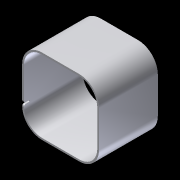
# Autodesk Inventor part: outer
Saved by Autodesk Inventor 2012 (Build 160160000, 160)
## iProperties
Created: 2012-11-10
Part Number: outer
Material: Default
Document SubType Name: Modeling
Designer: SONY
Density: 1 g/cm^3
Author: SONY
Autodesk Inventor part; units mm, degrees
ref_plane "YZ Plane" through (0, 0, 0) normal (1, 0, 0) x (0, 1, 0)
ref_plane "XZ Plane" through (0, 0, 0) normal (0, 1, 0) x (-1, 0, 0)
sketch "Sketch1" plane through (0, 0, 0) normal (0, 0, 1) x (1, 0, 0)
  arc A0 (37.77, -51.7625) -> (57.823, -30.1392) centre (37.77, -31.6525) ccw
  arc A1 (57.88, 4.9774) -> (37.77, 25.0874) centre (37.77, 4.9774) ccw
  arc A2 (-20.11, -31.6525) -> (0, -51.7625) centre (0, -31.6525) ccw
  arc A3 (0, 25.0874) -> (-20.11, 4.9774) centre (0, 4.9774) ccw
  line L0 (37.77, 25.0874) -> (0, 25.0874)
  line L1 (-20.11, -31.6525) -> (-20.11, 4.9774)
  line L2 (57.88, 4.9774) -> (57.88, -31.6525)
  line L3 (38.6468, -51.7625) -> (0, -51.7625)
  line L4 (27.06, -29.8525) -> (27.06, -31.6525) projected
  line L5 (20.48, -29.8525) -> (20.48, -31.8868) projected
  line L6 (5.94, -31.6525) -> (5.94, -29.8525) projected
  line L7 (12.52, -31.6525) -> (12.52, -29.8525) projected
  line L8 (1.8, -23.26) -> (0, -23.26) projected
  line L9 (1.8, -16.68) -> (0, -16.68) projected
  line L10 (0, -8.4695) -> (1.8, -8.4695) projected
  line L11 (0, -2.14) -> (1.8, -2.14) projected
  line L12 (37.77, 23.2874) -> (0, 23.2874) projected
  arc A4 (0, 23.2874) -> (-18.31, 4.9774) centre (0, 4.9774) ccw projected
  line L13 (-18.31, -31.6525) -> (-18.31, 4.9774) projected
  arc A5 (-18.31, -31.6525) -> (0, -49.9625) centre (0, -31.6525) ccw projected
  line L14 (37.77, -49.9625) -> (0, -49.9625) projected
  arc A6 (37.77, -49.9625) -> (56.08, -31.6525) centre (37.77, -31.6525) ccw projected
  line L15 (56.08, 4.9774) -> (56.08, -31.6525) projected
  arc A7 (56.08, 4.9774) -> (37.77, 23.2874) centre (37.77, 4.9774) ccw projected
  line L16 (20.48, -29.8525) -> (12.52, -29.8525) projected
  line L17 (12.52, -31.6525) -> (16.485, -31.6525) projected
  arc A8 (17.985, -33.1525) -> (16.485, -31.6525) centre (16.485, -33.1525) ccw projected
  line L18 (17.985, -36.5025) -> (17.985, -33.1525) projected
  arc A9 (16.485, -38.0025) -> (17.985, -36.5025) centre (16.485, -36.5025) ccw projected
  line L19 (0, -38.0025) -> (16.485, -38.0025) projected
  arc A10 (-1.669, -37.7792) -> (0, -38.0025) centre (0, -31.6525) ccw projected
  arc A11 (-2.3373, -35.2732) -> (-1.669, -37.7792) centre (-1.2747, -36.332) ccw projected
  line L20 (0.942, -31.9822) -> (-2.3373, -35.2732) projected
  arc A12 (2.3363, -31.5782) -> (0.942, -31.9822) centre (2.0045, -33.041) ccw projected
  arc A13 (2.3363, -31.5782) -> (3, -31.6525) centre (3, -28.6525) ccw projected
  line L21 (3, -31.6525) -> (5.94, -31.6525) projected
  line L22 (5.94, -29.8525) -> (4.3, -29.8525) projected
  arc A14 (1.8, -27.3525) -> (4.3, -29.8525) centre (4.3, -27.3525) ccw projected
  line L23 (1.8, -27.3525) -> (1.8, -23.26) projected
  line L24 (0, -28.6525) -> (0, -23.26) projected
  arc A15 (0, -28.6525) -> (0.0741, -29.315) centre (3, -28.6525) ccw projected
  arc A16 (-0.3264, -30.705) -> (0.0741, -29.315) centre (-1.3889, -29.6462) ccw projected
  line L25 (-3.6124, -34.0027) -> (-0.3264, -30.705) projected
  arc A17 (-6.1207, -33.3433) -> (-3.6124, -34.0027) centre (-4.6749, -32.9439) ccw projected
  arc A18 (-6.35, -31.6525) -> (-6.1207, -33.3433) centre (0, -31.6525) ccw projected
  line L26 (-6.35, -15.1) -> (-6.35, -31.6525) projected
  arc A19 (-4.85, -13.6) -> (-6.35, -15.1) centre (-4.85, -15.1) ccw projected
  line L27 (-1.5, -13.6) -> (-4.85, -13.6) projected
  arc A20 (0, -15.1) -> (-1.5, -13.6) centre (-1.5, -15.1) ccw projected
  line L28 (0, -16.68) -> (0, -15.1) projected
  line L29 (1.8, -16.68) -> (1.8, -8.4695) projected
  arc A21 (-1.5, -11.8) -> (0, -10.3) centre (-1.5, -10.3) ccw projected
  line L30 (-4.85, -11.8) -> (-1.5, -11.8) projected
  arc A22 (-6.35, -10.3) -> (-4.85, -11.8) centre (-4.85, -10.3) ccw projected
  line L31 (-6.35, 6.2525) -> (-6.35, -10.3) projected
  arc A23 (-6.1207, 7.9433) -> (-6.35, 6.2525) centre (0, 6.2525) ccw projected
  arc A24 (-3.6124, 8.6027) -> (-6.1207, 7.9433) centre (-4.6749, 7.5439) ccw projected
  line L32 (-0.3264, 5.305) -> (-3.6124, 8.6027) projected
  arc A25 (0.0741, 3.915) -> (-0.3264, 5.305) centre (-1.3889, 4.2462) ccw projected
  arc A26 (0.0741, 3.915) -> (0, 3.2525) centre (3, 3.2525) ccw projected
  line L33 (0, -2.14) -> (0, 3.2525) projected
  line L34 (1.8, -2.14) -> (1.8, 1.9525) projected
  arc A27 (4.3, 4.4525) -> (1.8, 1.9525) centre (4.3, 1.9525) ccw projected
  line L35 (4.3, 4.4525) -> (5.94, 4.4525) projected
  arc A28 (35.97, 1.9525) -> (33.47, 4.4525) centre (33.47, 1.9525) ccw projected
  line L36 (35.97, 1.9525) -> (35.97, -27.3525) projected
  arc A29 (33.47, -29.8525) -> (35.97, -27.3525) centre (33.47, -27.3525) ccw projected
  line L37 (33.47, -29.8525) -> (27.06, -29.8525) projected
  line L38 (27.06, -31.6525) -> (34.77, -31.6525) projected
  arc A30 (34.77, -31.6525) -> (35.4337, -31.5782) centre (34.77, -28.6525) ccw projected
  arc A31 (36.828, -31.9822) -> (35.4337, -31.5782) centre (35.7655, -33.041) ccw projected
  line L39 (40.1073, -35.2732) -> (36.828, -31.9822) projected
  arc A32 (39.439, -37.7792) -> (40.1073, -35.2732) centre (39.0447, -36.332) ccw projected
  arc A33 (37.77, -38.0025) -> (39.439, -37.7792) centre (37.77, -31.6525) ccw projected
  line L40 (21.285, -38.0025) -> (37.77, -38.0025) projected
  arc A34 (19.785, -36.5025) -> (21.285, -38.0025) centre (21.285, -36.5025) ccw projected
  line L41 (19.785, -33.1525) -> (19.785, -36.5025) projected
  arc A35 (20.48, -31.8868) -> (19.785, -33.1525) centre (21.285, -33.1525) ccw projected
  line L42 (37.77, 3.2525) -> (37.77, -10.3) projected
  arc A36 (37.77, 3.2525) -> (37.6959, 3.915) centre (34.77, 3.2525) ccw projected
  arc A37 (38.0964, 5.305) -> (37.6959, 3.915) centre (39.1589, 4.2462) ccw projected
  line L43 (41.3824, 8.6027) -> (38.0964, 5.305) projected
  arc A38 (43.8907, 7.9433) -> (41.3824, 8.6027) centre (42.4449, 7.5439) ccw projected
  arc A39 (44.12, 6.2525) -> (43.8907, 7.9433) centre (37.77, 6.2525) ccw projected
  line L44 (44.12, -10.3) -> (44.12, 6.2525) projected
  arc A40 (42.62, -11.8) -> (44.12, -10.3) centre (42.62, -10.3) ccw projected
  line L45 (39.27, -11.8) -> (42.62, -11.8) projected
  arc A41 (37.77, -10.3) -> (39.27, -11.8) centre (39.27, -10.3) ccw projected
  line L46 (44.12, -31.6525) -> (44.12, -15.1) projected
  arc A42 (43.8907, -33.3433) -> (44.12, -31.6525) centre (37.77, -31.6525) ccw projected
  arc A43 (41.3824, -34.0027) -> (43.8907, -33.3433) centre (42.4449, -32.9439) ccw projected
  line L47 (38.0964, -30.705) -> (41.3824, -34.0027) projected
  arc A44 (37.6959, -29.315) -> (38.0964, -30.705) centre (39.1589, -29.6462) ccw projected
  arc A45 (37.6959, -29.315) -> (37.77, -28.6525) centre (34.77, -28.6525) ccw projected
  line L48 (37.77, -15.1) -> (37.77, -28.6525) projected
  arc A46 (39.27, -13.6) -> (37.77, -15.1) centre (39.27, -15.1) ccw projected
  line L49 (42.62, -13.6) -> (39.27, -13.6) projected
  arc A47 (44.12, -15.1) -> (42.62, -13.6) centre (42.62, -15.1) ccw projected
  arc A48 (35.4337, 6.1782) -> (34.77, 6.2525) centre (34.77, 3.2525) ccw projected
  line L50 (16.485, 6.2525) -> (12.2695, 6.2525) projected
  arc A49 (19.785, 7.7525) -> (20.48, 6.4868) centre (21.285, 7.7525) ccw projected
  line L51 (19.785, 11.1025) -> (19.785, 7.7525) projected
  arc A50 (21.285, 12.6025) -> (19.785, 11.1025) centre (21.285, 11.1025) ccw projected
  line L52 (37.77, 12.6025) -> (21.285, 12.6025) projected
  arc A51 (39.439, 12.3792) -> (37.77, 12.6025) centre (37.77, 6.2525) ccw projected
  arc A52 (40.1073, 9.8732) -> (39.439, 12.3792) centre (39.0447, 10.932) ccw projected
  line L53 (36.828, 6.5822) -> (40.1073, 9.8732) projected
  arc A53 (35.4337, 6.1782) -> (36.828, 6.5822) centre (35.7655, 7.641) ccw projected
  arc A54 (-1.669, 12.3792) -> (-2.3373, 9.8732) centre (-1.2747, 10.932) ccw projected
  arc A55 (0, 12.6025) -> (-1.669, 12.3792) centre (0, 6.2525) ccw projected
  line L54 (16.485, 12.6025) -> (0, 12.6025) projected
  arc A56 (17.985, 11.1025) -> (16.485, 12.6025) centre (16.485, 11.1025) ccw projected
  line L55 (17.985, 7.7525) -> (17.985, 11.1025) projected
  arc A57 (16.485, 6.2525) -> (17.985, 7.7525) centre (16.485, 7.7525) ccw projected
  line L56 (5.94, 6.2525) -> (3, 6.2525) projected
  arc A58 (3, 6.2525) -> (2.3363, 6.1782) centre (3, 3.2525) ccw projected
  arc A59 (0.942, 6.5822) -> (2.3363, 6.1782) centre (2.0045, 7.641) ccw projected
  line L57 (-2.3373, 9.8732) -> (0.942, 6.5822) projected
  line L58 (0, -10.3) -> (0, -8.4695) projected
  line L59 (5.94, 4.4525) -> (5.94, 6.2525) projected
  line L60 (12.2695, 4.4525) -> (12.2695, 6.2525) projected
  line L61 (12.2695, 4.4525) -> (20.48, 4.4525) projected
  line L62 (20.48, 6.4868) -> (20.48, 4.4525) projected
  line L63 (34.77, 6.2525) -> (27.06, 6.2525) projected
  line L64 (27.06, 6.2525) -> (27.06, 4.4525) projected
  line L65 (27.06, 4.4525) -> (33.47, 4.4525) projected
  point P0 (0, 0)
  dimension "d52" = 1.8
  constraints: 9 point on circle, 8 end point, 8 tangent, 4 centre point, 4 coincident, 2 perpendicular, 1 parallel, 1 point on line
  measures "d52" distance between parallel lines of L13 L1
ref_plane "Work Plane1" through (-11.96, -43.6125, -59.69) normal (0, 0, -1) x (0, 1, 0)
extrude "Extrusion1" add sketch "Sketch1" against normal up to surface (59.69 mm away) contours L3 A2 L1 A3 L0 A1 L2 A0
sketch "Sketch4" plane through (37.77, -51.7625, -59.69) normal (0, 0, -1) x (-1, 0, 0)
  line L0 (27.885, 20.11) -> (27.885, 0)
  line L1 (27.885, 0) -> (9.885, 0)
  line L2 (9.885, 0) -> (9.885, 20.11)
  line L3 (37.77, 48.0625) -> (57.88, 48.0625)
  line L4 (57.88, 48.0625) -> (57.88, 30.0625)
  line L5 (57.88, 30.0625) -> (37.77, 30.0625)
  line L6 (27.885, 58.015) -> (27.885, 76.8499)
  line L7 (27.885, 76.8499) -> (9.885, 76.8499)
  line L8 (9.885, 76.8499) -> (9.885, 58.015)
  line L9 (-20.11, 48.0625) -> (0, 48.0625)
  line L10 (0, 30.0625) -> (-20.11, 30.0625)
  line L11 (-20.11, 30.0625) -> (-20.11, 48.0625)
  arc A0 (3, 58.015) -> (0, 55.015) centre (3, 55.015) ccw
  arc A1 (37.77, 55.015) -> (34.77, 58.015) centre (34.77, 55.015) ccw
  arc A2 (34.77, 20.11) -> (37.77, 23.11) centre (34.77, 23.11) ccw
  arc A3 (0, 23.11) -> (3, 20.11) centre (3, 23.11) ccw
  line L12 (0, 76.8499) -> (37.77, 76.8499) projected
  line L13 (3, 20.11) -> (9.885, 20.11)
  line L14 (0, 23.11) -> (0, 30.0625)
  line L15 (27.885, 20.11) -> (34.77, 20.11)
  line L16 (37.77, 23.11) -> (37.77, 30.0625)
  line L17 (37.77, 48.0625) -> (37.77, 55.015)
  line L18 (34.77, 58.015) -> (27.885, 58.015)
  line L19 (9.885, 58.015) -> (3, 58.015)
  line L20 (4.3, 21.91) -> (33.47, 21.91)
  arc A4 (33.47, 21.91) -> (35.97, 24.41) centre (33.47, 24.41) ccw
  line L21 (35.97, 24.41) -> (35.97, 34.0931)
  line L22 (35.97, 34.0931) -> (35.97, 53.715)
  arc A5 (35.97, 53.715) -> (33.47, 56.215) centre (33.47, 53.715) ccw
  line L23 (33.47, 56.215) -> (4.3, 56.215)
  arc A6 (4.3, 56.215) -> (1.8, 53.715) centre (4.3, 53.715) ccw
  line L24 (1.8, 53.715) -> (1.8, 41.6025)
  line L25 (1.8, 41.6025) -> (1.8, 24.41)
  arc A7 (1.8, 24.41) -> (4.3, 21.91) centre (4.3, 24.41) ccw
  line L26 (0, 55.015) -> (0, 48.0625)
  line L27 (-20.11, 20.11) -> (-20.11, 56.7399) projected
  line L28 (37.77, 0) -> (0, 0) projected
  line L29 (57.88, 56.7399) -> (57.88, 20.11) projected
  arc A8 (0.942, 58.3447) -> (2.3363, 57.9407) centre (2.0045, 59.4035) ccw projected
  line L30 (-2.3373, 61.6357) -> (0.942, 58.3447) projected
  arc A9 (-1.669, 64.1417) -> (-2.3373, 61.6357) centre (-1.2747, 62.6945) ccw projected
  arc A10 (0, 64.365) -> (-1.669, 64.1417) centre (0, 58.015) ccw projected
  line L31 (16.485, 64.365) -> (0, 64.365) projected
  arc A11 (17.985, 62.865) -> (16.485, 64.365) centre (16.485, 62.865) ccw projected
  line L32 (17.985, 59.515) -> (17.985, 62.865) projected
  arc A12 (16.485, 58.015) -> (17.985, 59.515) centre (16.485, 59.515) ccw projected
  line L33 (3, 58.015) -> (16.485, 58.015) projected
  arc A13 (3, 58.015) -> (2.3363, 57.9407) centre (3, 55.015) ccw projected
  arc A14 (35.97, 53.715) -> (33.47, 56.215) centre (33.47, 53.715) ccw projected
  line L34 (35.97, 24.41) -> (35.97, 53.715) projected
  arc A15 (33.47, 21.91) -> (35.97, 24.41) centre (33.47, 24.41) ccw projected
  line L35 (4.3, 21.91) -> (33.47, 21.91) projected
  arc A16 (1.8, 24.41) -> (4.3, 21.91) centre (4.3, 24.41) ccw projected
  line L36 (1.8, 53.715) -> (1.8, 24.41) projected
  arc A17 (4.3, 56.215) -> (1.8, 53.715) centre (4.3, 53.715) ccw projected
  line L37 (33.47, 56.215) -> (4.3, 56.215) projected
  arc A18 (-1.5, 39.9625) -> (0, 41.4625) centre (-1.5, 41.4625) ccw projected
  line L38 (-4.85, 39.9625) -> (-1.5, 39.9625) projected
  arc A19 (-6.35, 41.4625) -> (-4.85, 39.9625) centre (-4.85, 41.4625) ccw projected
  line L39 (-6.35, 58.015) -> (-6.35, 41.4625) projected
  arc A20 (-6.1207, 59.7058) -> (-6.35, 58.015) centre (0, 58.015) ccw projected
  arc A21 (-3.6124, 60.3652) -> (-6.1207, 59.7058) centre (-4.6749, 59.3064) ccw projected
  line L40 (-0.3264, 57.0675) -> (-3.6124, 60.3652) projected
  arc A22 (0.0741, 55.6775) -> (-0.3264, 57.0675) centre (-1.3889, 56.0087) ccw projected
  arc A23 (0.0741, 55.6775) -> (0, 55.015) centre (3, 55.015) ccw projected
  line L41 (0, 41.4625) -> (0, 55.015) projected
  arc A24 (39.27, 38.1625) -> (37.77, 36.6625) centre (39.27, 36.6625) ccw projected
  line L42 (42.62, 38.1625) -> (39.27, 38.1625) projected
  arc A25 (44.12, 36.6625) -> (42.62, 38.1625) centre (42.62, 36.6625) ccw projected
  line L43 (44.12, 20.11) -> (44.12, 36.6625) projected
  arc A26 (43.8907, 18.4192) -> (44.12, 20.11) centre (37.77, 20.11) ccw projected
  arc A27 (41.3824, 17.7598) -> (43.8907, 18.4192) centre (42.4449, 18.8186) ccw projected
  line L44 (38.0964, 21.0575) -> (41.3824, 17.7598) projected
  arc A28 (37.6959, 22.4475) -> (38.0964, 21.0575) centre (39.1589, 22.1163) ccw projected
  arc A29 (37.6959, 22.4475) -> (37.77, 23.11) centre (34.77, 23.11) ccw projected
  line L45 (37.77, 36.6625) -> (37.77, 23.11) projected
  arc A30 (0, 36.6625) -> (-1.5, 38.1625) centre (-1.5, 36.6625) ccw projected
  line L46 (0, 23.11) -> (0, 36.6625) projected
  arc A31 (0, 23.11) -> (0.0741, 22.4475) centre (3, 23.11) ccw projected
  arc A32 (-0.3264, 21.0575) -> (0.0741, 22.4475) centre (-1.3889, 22.1163) ccw projected
  line L47 (-3.6124, 17.7598) -> (-0.3264, 21.0575) projected
  arc A33 (-6.1207, 18.4192) -> (-3.6124, 17.7598) centre (-4.6749, 18.8186) ccw projected
  arc A34 (-6.35, 20.11) -> (-6.1207, 18.4192) centre (0, 20.11) ccw projected
  line L48 (-6.35, 36.6625) -> (-6.35, 20.11) projected
  arc A35 (-4.85, 38.1625) -> (-6.35, 36.6625) centre (-4.85, 36.6625) ccw projected
  line L49 (-1.5, 38.1625) -> (-4.85, 38.1625) projected
  arc A36 (38.0964, 57.0675) -> (37.6959, 55.6775) centre (39.1589, 56.0087) ccw projected
  line L50 (41.3824, 60.3652) -> (38.0964, 57.0675) projected
  arc A37 (43.8907, 59.7058) -> (41.3824, 60.3652) centre (42.4449, 59.3064) ccw projected
  arc A38 (44.12, 58.015) -> (43.8907, 59.7058) centre (37.77, 58.015) ccw projected
  line L51 (44.12, 41.4625) -> (44.12, 58.015) projected
  arc A39 (42.62, 39.9625) -> (44.12, 41.4625) centre (42.62, 41.4625) ccw projected
  line L52 (39.27, 39.9625) -> (42.62, 39.9625) projected
  arc A40 (37.77, 41.4625) -> (39.27, 39.9625) centre (39.27, 41.4625) ccw projected
  line L53 (37.77, 55.015) -> (37.77, 41.4625) projected
  arc A41 (37.77, 55.015) -> (37.6959, 55.6775) centre (34.77, 55.015) ccw projected
  arc A42 (35.4337, 57.9407) -> (36.828, 58.3447) centre (35.7655, 59.4035) ccw projected
  arc A43 (35.4337, 57.9407) -> (34.77, 58.015) centre (34.77, 55.015) ccw projected
  line L54 (21.285, 58.015) -> (34.77, 58.015) projected
  arc A44 (19.785, 59.515) -> (21.285, 58.015) centre (21.285, 59.515) ccw projected
  line L55 (19.785, 62.865) -> (19.785, 59.515) projected
  arc A45 (21.285, 64.365) -> (19.785, 62.865) centre (21.285, 62.865) ccw projected
  line L56 (37.77, 64.365) -> (21.285, 64.365) projected
  arc A46 (39.439, 64.1417) -> (37.77, 64.365) centre (37.77, 58.015) ccw projected
  arc A47 (40.1073, 61.6357) -> (39.439, 64.1417) centre (39.0447, 62.6945) ccw projected
  line L57 (36.828, 58.3447) -> (40.1073, 61.6357) projected
  arc A48 (17.985, 18.61) -> (16.485, 20.11) centre (16.485, 18.61) ccw projected
  line L58 (17.985, 15.26) -> (17.985, 18.61) projected
  arc A49 (16.485, 13.76) -> (17.985, 15.26) centre (16.485, 15.26) ccw projected
  line L59 (0, 13.76) -> (16.485, 13.76) projected
  arc A50 (-1.669, 13.9833) -> (0, 13.76) centre (0, 20.11) ccw projected
  arc A51 (-2.3373, 16.4893) -> (-1.669, 13.9833) centre (-1.2747, 15.4305) ccw projected
  line L60 (0.942, 19.7803) -> (-2.3373, 16.4893) projected
  arc A52 (2.3363, 20.1843) -> (0.942, 19.7803) centre (2.0045, 18.7215) ccw projected
  arc A53 (2.3363, 20.1843) -> (3, 20.11) centre (3, 23.11) ccw projected
  line L61 (16.485, 20.11) -> (3, 20.11) projected
  arc A54 (36.828, 19.7803) -> (35.4337, 20.1843) centre (35.7655, 18.7215) ccw projected
  line L62 (40.1073, 16.4893) -> (36.828, 19.7803) projected
  arc A55 (39.439, 13.9833) -> (40.1073, 16.4893) centre (39.0447, 15.4305) ccw projected
  arc A56 (37.77, 13.76) -> (39.439, 13.9833) centre (37.77, 20.11) ccw projected
  line L63 (21.285, 13.76) -> (37.77, 13.76) projected
  arc A57 (19.785, 15.26) -> (21.285, 13.76) centre (21.285, 15.26) ccw projected
  line L64 (19.785, 18.61) -> (19.785, 15.26) projected
  arc A58 (21.285, 20.11) -> (19.785, 18.61) centre (21.285, 18.61) ccw projected
  line L65 (34.77, 20.11) -> (21.285, 20.11) projected
  arc A59 (34.77, 20.11) -> (35.4337, 20.1843) centre (34.77, 23.11) ccw projected
  arc A60 (0, 66.165) -> (-8.15, 58.015) centre (0, 58.015) ccw projected
  line L66 (-8.15, 20.11) -> (-8.15, 58.015) projected
  arc A61 (-8.15, 20.11) -> (0, 11.96) centre (0, 20.11) ccw projected
  line L67 (37.77, 11.96) -> (0, 11.96) projected
  arc A62 (37.77, 11.96) -> (45.92, 20.11) centre (37.77, 20.11) ccw projected
  line L68 (45.92, 58.015) -> (45.92, 20.11) projected
  arc A63 (45.92, 58.015) -> (37.77, 66.165) centre (37.77, 58.015) ccw projected
  line L69 (0, 66.165) -> (37.77, 66.165) projected
  point P0 (37.77, 51.7625)
  dimension "d58" = 18
  dimension "d59" = 8.1
  dimension "d60" = 18
  dimension "d61" = 8.1
  constraints: 52 end point, 24 collinear, 16 point on circle, 14 tangent, 8 centre point, 8 coincident, 5 parallel, 4 perpendicular, 2 horizontal
  measures "d58" distance of L10.end L9.start
  measures "d59" distance between parallel lines of L38 L9
  measures "d60" distance of L0.end L1.end
  measures "d61" distance between parallel lines of L58 L2
extrude "Extrusion4" add sketch "Sketch4" against normal blind 1.8 contours L65 A58 L64 A57 L63 L0 L67 L2 L59 A49 L58 A48 L61 L13 A3 L14 L46 A30 L49 A35 L48 L10 L66 L9 L39 A19 L38 A18 L41 L26 A0 L19 L33 A12 L32 A11 L31 L8 L69 L6 L56 A45 L55 A44 L54 L18 A1 L17 L53 A40 L52 A39 L51 L3 L68 L5 L43 A25 L42 A24 L45 L16 A2 L15 | L0 L63 A57 L64 A58 L65 | L0 L1 L2 L67 | L2 L61 A48 L58 A49 L59 | L68 L3 L4 L5 | L45 A24 L42 A25 L43 L5 | L10 L11 L9 L66 | L51 A39 L52 A40 L53 L3 | L48 A35 L49 A30 L46 L10 | L9 L41 A18 L38 A19 L39 | L69 L8 L7 L6 | L6 L54 A44 L55 A45 L56 | L31 A11 L32 A12 L33 L8
fillet "Fillet2" radius 3.175 8 edges at (37.77, -21.7, -58.79) (27.885, -31.6525, -58.79) (9.885, -31.6525, -58.79) (0, -21.7, -58.79) (0, -3.7, -58.79) (9.885, 6.2525, -58.79) (37.77, -3.7, -58.79) (27.885, 6.2525, -58.79)
sketch "Sketch5" plane through (37.77, -51.7625, -57.89) normal (0, 0, 1) x (1, 0, 0)
  line L0 (-56.08, 48.0625) -> (-40.945, 48.0625) projected
  line L1 (-40.945, 30.0625) -> (-56.08, 30.0625) projected
  line L2 (-43.82, 34.0625) -> (-38.07, 34.0625)
  line L3 (-38.07, 34.0625) -> (-38.07, 30.0625)
  line L4 (-38.07, 30.0625) -> (-43.82, 30.0625)
  line L5 (-43.82, 30.0625) -> (-43.82, 34.0625)
  line L6 (-43.82, 48.0625) -> (-38.07, 48.0625)
  line L7 (-38.07, 48.0625) -> (-38.07, 44.0625)
  line L8 (-38.07, 44.0625) -> (-43.82, 44.0625)
  line L9 (-43.82, 44.0625) -> (-43.82, 48.0625)
  line L10 (-13.885, 14.1275) -> (-13.885, 19.8775)
  line L11 (-13.885, 19.8775) -> (-9.885, 19.8775)
  line L12 (-9.885, 19.8775) -> (-9.885, 14.1275)
  line L13 (-9.885, 14.1275) -> (-13.885, 14.1275)
  line L14 (-27.885, 14.1275) -> (-27.885, 19.8775)
  line L15 (-27.885, 19.8775) -> (-23.885, 19.8775)
  line L16 (-23.885, 19.8775) -> (-23.885, 14.1275)
  line L17 (-23.885, 14.1275) -> (-27.885, 14.1275)
  line L18 (6.05, 44.0625) -> (0.3, 44.0625)
  line L19 (0.3, 44.0625) -> (0.3, 48.0625)
  line L20 (0.3, 48.0625) -> (6.05, 48.0625)
  line L21 (6.05, 48.0625) -> (6.05, 44.0625)
  line L22 (6.05, 30.0625) -> (0.3, 30.0625)
  line L23 (0.3, 30.0625) -> (0.3, 34.0625)
  line L24 (0.3, 34.0625) -> (6.05, 34.0625)
  line L25 (6.05, 34.0625) -> (6.05, 30.0625)
  line L26 (-23.885, 63.9975) -> (-23.885, 58.2475)
  line L27 (-23.885, 58.2475) -> (-27.885, 58.2475)
  line L28 (-27.885, 58.2475) -> (-27.885, 63.9975)
  line L29 (-27.885, 63.9975) -> (-23.885, 63.9975)
  line L30 (-9.885, 63.9975) -> (-9.885, 58.2475)
  line L31 (-9.885, 58.2475) -> (-13.885, 58.2475)
  line L32 (-13.885, 58.2475) -> (-13.885, 63.9975)
  line L33 (-13.885, 63.9975) -> (-9.885, 63.9975)
  line L34 (3.175, 48.0625) -> (18.31, 48.0625) projected
  line L35 (-17.29, 23.18) -> (-17.29, 21.1457) projected
  line L36 (-17.29, 23.18) -> (-25.25, 23.18) projected
  line L37 (-25.25, 21.38) -> (-25.25, 23.18) projected
  line L38 (-25.25, 21.38) -> (-21.285, 21.38) projected
  arc A0 (-19.785, 19.88) -> (-21.285, 21.38) centre (-21.285, 19.88) ccw projected
  line L39 (-19.785, 16.53) -> (-19.785, 19.88) projected
  arc A1 (-21.285, 15.03) -> (-19.785, 16.53) centre (-21.285, 16.53) ccw projected
  line L40 (-37.77, 15.03) -> (-21.285, 15.03) projected
  arc A2 (-39.439, 15.2533) -> (-37.77, 15.03) centre (-37.77, 21.38) ccw projected
  arc A3 (-40.1073, 17.7593) -> (-39.439, 15.2533) centre (-39.0447, 16.7005) ccw projected
  line L41 (-36.828, 21.0503) -> (-40.1073, 17.7593) projected
  arc A4 (-35.4337, 21.4543) -> (-36.828, 21.0503) centre (-35.7655, 19.9915) ccw projected
  arc A5 (-35.4337, 21.4543) -> (-34.77, 20.11) centre (-34.77, 24.38) ccw projected
  line L42 (-34.77, 21.38) -> (-31.83, 21.38) projected
  line L43 (-31.83, 21.38) -> (-31.83, 23.18) projected
  line L44 (-31.83, 23.18) -> (-33.47, 23.18) projected
  arc A6 (-35.97, 24.41) -> (-33.47, 21.91) centre (-33.47, 25.68) ccw projected
  line L45 (-35.97, 24.41) -> (-35.97, 29.7725) projected
  line L46 (-35.97, 29.7725) -> (-37.77, 29.7725) projected
  line L47 (-37.77, 23.11) -> (-37.77, 29.7725) projected
  arc A7 (-37.77, 23.11) -> (-37.6959, 23.7175) centre (-34.77, 24.38) ccw projected
  arc A8 (-38.0964, 22.3275) -> (-37.6959, 23.7175) centre (-39.1589, 23.3863) ccw projected
  line L48 (-41.3824, 19.0298) -> (-38.0964, 22.3275) projected
  arc A9 (-43.8907, 19.6892) -> (-41.3824, 19.0298) centre (-42.4449, 20.0886) ccw projected
  arc A10 (-44.12, 21.38) -> (-43.8907, 19.6892) centre (-37.77, 21.38) ccw projected
  line L49 (-44.12, 37.9325) -> (-44.12, 21.38) projected
  arc A11 (-42.62, 39.4325) -> (-44.12, 37.9325) centre (-42.62, 37.9325) ccw projected
  line L50 (-39.27, 39.4325) -> (-42.62, 39.4325) projected
  arc A12 (-37.77, 37.9325) -> (-39.27, 39.4325) centre (-39.27, 37.9325) ccw projected
  line L51 (-37.77, 36.3525) -> (-37.77, 37.9325) projected
  line L52 (-35.97, 36.3525) -> (-37.77, 36.3525) projected
  line L53 (-35.97, 36.3525) -> (-35.97, 44.563) projected
  line L54 (-37.77, 44.563) -> (-35.97, 44.563) projected
  line L55 (-37.77, 42.7325) -> (-37.77, 44.563) projected
  arc A13 (-39.27, 41.2325) -> (-37.77, 42.7325) centre (-39.27, 42.7325) ccw projected
  line L56 (-42.62, 41.2325) -> (-39.27, 41.2325) projected
  arc A14 (-44.12, 42.7325) -> (-42.62, 41.2325) centre (-42.62, 42.7325) ccw projected
  line L57 (-44.12, 59.285) -> (-44.12, 42.7325) projected
  arc A15 (-43.8907, 60.9758) -> (-44.12, 59.285) centre (-37.77, 59.285) ccw projected
  arc A16 (-41.3824, 61.6352) -> (-43.8907, 60.9758) centre (-42.4449, 60.5764) ccw projected
  line L58 (-38.0964, 58.3375) -> (-41.3824, 61.6352) projected
  arc A17 (-37.6959, 56.9475) -> (-38.0964, 58.3375) centre (-39.1589, 57.2787) ccw projected
  arc A18 (-37.6959, 56.9475) -> (-37.77, 55.015) centre (-34.77, 56.285) ccw projected
  line L59 (-37.77, 50.8925) -> (-37.77, 55.015) projected
  line L60 (-37.77, 50.8925) -> (-35.97, 50.8925) projected
  line L61 (-35.97, 50.8925) -> (-35.97, 53.715) projected
  arc A19 (-33.47, 56.215) -> (-35.97, 53.715) centre (-33.47, 54.985) ccw projected
  line L62 (-33.47, 57.485) -> (-31.83, 57.485) projected
  line L63 (-31.83, 57.485) -> (-31.83, 59.285) projected
  line L64 (-31.83, 59.285) -> (-34.77, 59.285) projected
  arc A20 (-34.77, 58.015) -> (-35.4337, 59.2107) centre (-34.77, 56.285) ccw projected
  arc A21 (-36.828, 59.6147) -> (-35.4337, 59.2107) centre (-35.7655, 60.6735) ccw projected
  line L65 (-40.1073, 62.9057) -> (-36.828, 59.6147) projected
  arc A22 (-39.439, 65.4117) -> (-40.1073, 62.9057) centre (-39.0447, 63.9645) ccw projected
  arc A23 (-37.77, 65.635) -> (-39.439, 65.4117) centre (-37.77, 59.285) ccw projected
  line L66 (-21.285, 65.635) -> (-37.77, 65.635) projected
  arc A24 (-19.785, 64.135) -> (-21.285, 65.635) centre (-21.285, 64.135) ccw projected
  line L67 (-19.785, 60.785) -> (-19.785, 64.135) projected
  arc A25 (-21.285, 59.285) -> (-19.785, 60.785) centre (-21.285, 60.785) ccw projected
  line L68 (-21.285, 59.285) -> (-25.5005, 59.285) projected
  line L69 (-25.5005, 57.485) -> (-25.5005, 59.285) projected
  line L70 (-25.5005, 57.485) -> (-17.29, 57.485) projected
  line L71 (-17.29, 59.5193) -> (-17.29, 57.485) projected
  arc A26 (-17.985, 60.785) -> (-17.29, 59.5193) centre (-16.485, 60.785) ccw projected
  line L72 (-17.985, 64.135) -> (-17.985, 60.785) projected
  arc A27 (-16.485, 65.635) -> (-17.985, 64.135) centre (-16.485, 64.135) ccw projected
  line L73 (0, 65.635) -> (-16.485, 65.635) projected
  arc A28 (1.669, 65.4117) -> (0, 65.635) centre (0, 59.285) ccw projected
  arc A29 (2.3373, 62.9057) -> (1.669, 65.4117) centre (1.2747, 63.9645) ccw projected
  line L74 (-0.942, 59.6147) -> (2.3373, 62.9057) projected
  arc A30 (-2.3363, 59.2107) -> (-0.942, 59.6147) centre (-2.0045, 60.6735) ccw projected
  arc A31 (-2.3363, 59.2107) -> (-3, 58.015) centre (-3, 56.285) ccw projected
  line L75 (-3, 59.285) -> (-10.71, 59.285) projected
  line L76 (-10.71, 59.285) -> (-10.71, 57.485) projected
  line L77 (-10.71, 57.485) -> (-4.3, 57.485) projected
  arc A32 (-1.8, 53.715) -> (-4.3, 56.215) centre (-4.3, 54.985) ccw projected
  line L78 (-1.8, 53.715) -> (-1.8, 24.41) projected
  arc A33 (-4.3, 21.91) -> (-1.8, 24.41) centre (-4.3, 25.68) ccw projected
  line L79 (-4.3, 23.18) -> (-10.71, 23.18) projected
  line L80 (-10.71, 23.18) -> (-10.71, 21.38) projected
  line L81 (-10.71, 21.38) -> (-3, 21.38) projected
  arc A34 (-3, 20.11) -> (-2.3363, 21.4543) centre (-3, 24.38) ccw projected
  arc A35 (-0.942, 21.0503) -> (-2.3363, 21.4543) centre (-2.0045, 19.9915) ccw projected
  line L82 (2.3373, 17.7593) -> (-0.942, 21.0503) projected
  arc A36 (1.669, 15.2533) -> (2.3373, 17.7593) centre (1.2747, 16.7005) ccw projected
  arc A37 (0, 15.03) -> (1.669, 15.2533) centre (0, 21.38) ccw projected
  line L83 (-16.485, 15.03) -> (0, 15.03) projected
  arc A38 (-17.985, 16.53) -> (-16.485, 15.03) centre (-16.485, 16.53) ccw projected
  line L84 (-17.985, 19.88) -> (-17.985, 16.53) projected
  arc A39 (-17.29, 21.1457) -> (-17.985, 19.88) centre (-16.485, 19.88) ccw projected
  line L85 (6.35, 21.38) -> (6.35, 37.9325) projected
  arc A40 (6.1207, 19.6892) -> (6.35, 21.38) centre (0, 21.38) ccw projected
  arc A41 (3.6124, 19.0298) -> (6.1207, 19.6892) centre (4.6749, 20.0886) ccw projected
  line L86 (0.3264, 22.3275) -> (3.6124, 19.0298) projected
  arc A42 (-0.0741, 23.7175) -> (0.3264, 22.3275) centre (1.3889, 23.3863) ccw projected
  arc A43 (-0.0741, 23.7175) -> (0, 23.11) centre (-3, 24.38) ccw projected
  line L87 (0, 37.9325) -> (0, 23.11) projected
  arc A44 (1.5, 39.4325) -> (0, 37.9325) centre (1.5, 37.9325) ccw projected
  line L88 (4.85, 39.4325) -> (1.5, 39.4325) projected
  arc A45 (6.35, 37.9325) -> (4.85, 39.4325) centre (4.85, 37.9325) ccw projected
  line L89 (0, 55.015) -> (0, 42.7325) projected
  arc A46 (0, 55.015) -> (-0.0741, 56.9475) centre (-3, 56.285) ccw projected
  arc A47 (0.3264, 58.3375) -> (-0.0741, 56.9475) centre (1.3889, 57.2787) ccw projected
  line L90 (3.6124, 61.6352) -> (0.3264, 58.3375) projected
  arc A48 (6.1207, 60.9758) -> (3.6124, 61.6352) centre (4.6749, 60.5764) ccw projected
  arc A49 (6.35, 59.285) -> (6.1207, 60.9758) centre (0, 59.285) ccw projected
  line L91 (6.35, 42.7325) -> (6.35, 59.285) projected
  arc A50 (4.85, 41.2325) -> (6.35, 42.7325) centre (4.85, 42.7325) ccw projected
  line L92 (1.5, 41.2325) -> (4.85, 41.2325) projected
  arc A51 (0, 42.7325) -> (1.5, 41.2325) centre (1.5, 42.7325) ccw projected
  line L93 (0, 77.5899) -> (-37.77, 77.5899) projected
  arc A52 (-37.77, 77.5899) -> (-57.35, 58.0099) centre (-37.77, 58.0099) ccw projected
  line L94 (-57.35, 58.0099) -> (-57.35, 21.38) projected
  arc A53 (-57.35, 21.38) -> (-37.77, 1.8) centre (-37.77, 21.38) ccw projected
  line L95 (-37.77, 1.8) -> (0, 1.8) projected
  arc A54 (0, 1.8) -> (19.58, 21.38) centre (0, 21.38) ccw projected
  line L96 (19.58, 21.38) -> (19.58, 58.0099) projected
  arc A55 (19.58, 58.0099) -> (0, 77.5899) centre (0, 58.0099) ccw projected
  point P0 (-55.445, 32.7025)
  point P1 (-37.77, 51.7625)
  point P2 (-18.885, 39.0625)
  point P3 (-21.285, 22.42)
  point P4 (-3, 26.92)
  point P5 (17.675, 50.5025)
  point P6 (-37.77, 50.5025)
  point P7 (-37.77, 32.7025)
  point P8 (-56.08, 30.0625)
  point P9 (18.31, 48.0625)
  point P10 (-40.945, 48.0625)
  dimension "d40" = 360
  dimension "d53" = 4
  dimension "d54" = 4
  dimension "d62" = 0.3
  dimension "d63" = 0.3
  dimension "d64" = 0.3
  constraints: 64 end point, 5 horizontal, 4 parallel, 2 collinear, 2 perpendicular, 88 other
  measures "d53" distance of L4.end L2.start
  measures "d54" distance of L8.end L6.start
  measures "d62" distance between parallel lines of L57 L9
  measures "d63" distance between parallel lines of L55 L3
  measures "d64" distance between parallel lines of L89 L19
extrude "Extrusion5" add sketch "Sketch5" along normal blind 1.8 contours L0 L6 L7 L8 L9 | L1 L5 L2 L3 L4 | L10 L83 L12 L13 | L10 L11 L12 L83 | L14 L40 L16 L17 | L14 L15 L16 L40 | L18 L19 L20 L21 | L22 L23 L24 L25 | L26 L68 L69 L27 L28 L29 | L26 L27 L69 L68 | L30 L75 L76 L31 L32 L33 | L30 L31 L76 L75
fillet "Fillet3" radius 0.5 38 edges at (-0.3, -19.7, -56.09) (-0.3, -17.7, -56.99) (-6.05, -19.7, -56.09) (-6.05, -17.7, -56.99) (-3.175, -17.7, -56.09) (-0.3, -5.7, -56.09) (-0.3, -7.7, -56.99) (-3.175, -7.7, -56.09) (-6.05, -7.7, -56.99) (-6.05, -5.7, -56.09) (43.82, -5.7, -56.09) (43.82, -7.7, -56.99) (40.945, -7.7, -56.09) (38.07, -7.7, -56.99) (38.07, -5.7, -56.09) (38.07, -19.7, -56.09) (38.07, -17.7, -56.99) (40.945, -17.7, -56.09) (43.82, -17.7, -56.99) (43.82, -19.7, -56.09) (25.885, 6.485, -56.09) (23.885, 9.36, -56.09) (23.885, 12.235, -56.99) (25.885, 12.235, -56.09) (11.885, 12.235, -56.09) (13.885, 12.235, -56.99) (13.885, 9.36, -56.09) (13.885, 6.485, -56.99) (11.885, 6.485, -56.09) (25.885, -37.635, -56.09) (23.885, -37.635, -56.99) (23.885, -34.76, -56.09) (25.885, -31.885, -56.09) (11.885, -31.885, -56.09) (13.885, -31.885, -56.99) (13.885, -34.76, -56.09) (13.885, -37.635, -56.99) (11.885, -37.635, -56.09)
sketch "Sketch6" plane through (-20.11, -31.6525, 0) normal (-1, 0, 0) x (0, 0, 1)
  line L0 (0, 36.6299) -> (0, 0) projected
  circle A0 centre (-5, 2.315) radius 0.75
  line L1 (-5, 3.065) -> (0, 3.065)
  line L2 (-5, 1.565) -> (0, 1.565)
  point P0 (0, 31.6525)
  point P1 (0, 18.315)
  dimension "d45" = 1.5
  dimension "d46" = 16
  dimension "d47" = 5
  constraints: 4 end point, 2 point on circle, 2 point on line, 2 tangent, 1 centre point, 1 midpoint, 1 parallel, 1 perpendicular
  measures "d45" diameter of A0
  measures "d46" vertical distance of point (0, 18.315) A0.centre
  measures "d47" distance from line of A0.centre L0
extrude "Extrusion6" cut sketch "Sketch6" against normal blind 1.8
fillet "Fillet4" radius 2 2 edges at (-19.21, -30.0875, 0) (-19.21, -28.5875, 0)
equation "\"d52\" = d0"
equation "\"d31\" = d0"
equation "\"d42\" = d0"
equation "\"d48\" = d0"
equation "\"d0\" = 1.8"
body "Solid1"
